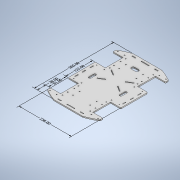
# Autodesk Inventor part: 底板2
Saved by Autodesk Inventor 2020.3 (Build 243373000, 373)
## iProperties
Created: 2020-12-02
Part Number: 底板2
Material: 常规
Document SubType Name: Sheet Metal
Designer: huang
Density: 1 g/cm^3
Sheet Metal Rule: 默认_mm
Appearance: 默认
Author: huang
Autodesk Inventor part; units mm, degrees
ref_plane "YZ Plane" through (0, 0, 0) normal (1, 0, 0) x (0, 1, 0)
ref_plane "XZ Plane" through (0, 0, 0) normal (0, 1, 0) x (-1, 0, 0)
ref_plane "XY Plane" through (0, 0, 0) normal (0, 0, 1) x (1, 0, 0)
sketch "草图1" plane through (0, 0, 0) normal (0, 1, 0) x (-1, 0, 0)
  line L0 (-53.8986, 0) -> (-183.8986, 0)
  line L1 (-237.8986, 27.6517) -> (-237.8986, 332.3483)
  line L2 (-183.8986, 360) -> (-53.8986, 360)
  line L3 (0.1014, 332.3483) -> (0.1014, 27.6517)
  arc A0 (-53.8986, 0) -> (-2.4158, 23.3117) centre (-151.1817, 283.3499) ccw
  arc A1 (-2.4158, 23.3117) -> (0.1014, 27.6517) centre (-4.8986, 27.6517) ccw
  arc A2 (-235.3815, 23.3117) -> (-183.8986, 0) centre (-86.6156, 283.3499) ccw
  arc A3 (-237.8986, 27.6517) -> (-235.3815, 23.3117) centre (-232.8986, 27.6517) ccw
  arc A4 (-2.4158, 336.6883) -> (-53.8986, 360) centre (-151.1817, 76.6501) ccw
  arc A5 (0.1014, 332.3483) -> (-2.4158, 336.6883) centre (-4.8986, 332.3483) ccw
  arc A6 (-183.8986, 360) -> (-235.3815, 336.6883) centre (-86.6156, 76.6501) ccw
  arc A7 (-235.3815, 336.6883) -> (-237.8986, 332.3483) centre (-232.8986, 332.3483) ccw
  line L4 (-118.8986, 10) -> (-135.3986, 10)
  line L5 (-118.8986, 10) -> (-102.3986, 10)
  line L6 (-102.3986, 13) -> (-135.3986, 13)
  arc A8 (-102.3986, 10) -> (-102.3986, 13) centre (-102.3986, 11.5) ccw
  arc A9 (-135.3986, 13) -> (-135.3986, 10) centre (-135.3986, 11.5) ccw
  arc A10 (-163.3986, 10) -> (-163.3986, 13) centre (-163.3986, 11.5) ccw
  line L7 (-163.3986, 10) -> (-176.3986, 10)
  line L8 (-176.3986, 13) -> (-163.3986, 13)
  arc A11 (-176.3986, 13) -> (-176.3986, 10) centre (-176.3986, 11.5) ccw
  line L9 (-118.8986, 50) -> (-127.3986, 50)
  line L10 (-118.8986, 50) -> (-110.3986, 50)
  line L11 (-110.3986, 65) -> (-127.3986, 65)
  arc A12 (-110.3986, 50) -> (-110.3986, 65) centre (-110.3986, 57.5) ccw
  arc A13 (-127.3986, 65) -> (-127.3986, 50) centre (-127.3986, 57.5) ccw
  circle A14 centre (-181.8986, 37) radius 2
  circle A15 centre (-197.8986, 26) radius 2
  circle A16 centre (-227.8986, 26) radius 2
  circle A17 centre (-181.8986, 109) radius 2
  circle A18 centre (-186.8986, 128) radius 2
  circle A19 centre (-222.3986, 128) radius 1.5
  arc A20 (-170.3606, 115.4419) -> (-168.7656, 112.901) centre (-169.5632, 114.1714) ccw
  arc A21 (-146.0526, 127.161) -> (-147.6449, 129.6982) centre (-146.7796, 128.473) ccw
  line L12 (-145.9139, 127.248) -> (-168.7656, 112.901)
  line L13 (-147.5067, 129.785) -> (-170.3606, 115.4419)
  arc A22 (-168.7665, 179.0438) -> (-170.3606, 176.5041) centre (-169.5635, 177.774) ccw
  arc A23 (-147.6449, 162.2478) -> (-146.0526, 164.785) centre (-146.7796, 163.473) ccw
  line L14 (-145.914, 164.698) -> (-168.7665, 179.0438)
  line L15 (-147.5067, 162.161) -> (-170.3606, 176.5041)
  arc A24 (-69.0307, 112.9022) -> (-67.4366, 115.4419) centre (-68.2337, 114.172) ccw
  arc A25 (-90.1523, 129.6982) -> (-91.7447, 127.161) centre (-91.0176, 128.473) ccw
  line L16 (-91.8832, 127.248) -> (-69.0307, 112.9022)
  line L17 (-90.2906, 129.785) -> (-67.4366, 115.4419)
  arc A26 (-91.7447, 164.785) -> (-90.1523, 162.2478) centre (-91.0176, 163.473) ccw
  line L18 (-90.2906, 162.161) -> (-67.4366, 176.5041)
  line L19 (-91.8832, 164.698) -> (-69.0307, 179.0438)
  arc A27 (-67.4366, 176.5041) -> (-69.0307, 179.0438) centre (-68.2337, 177.774) ccw
  arc A28 (-228.4486, 139.55) -> (-225.4486, 139.55) centre (-226.9486, 139.55) ccw
  line L20 (-225.4486, 139.55) -> (-225.4486, 151.55)
  line L21 (-228.4486, 151.55) -> (-228.4486, 139.55)
  arc A29 (-225.4486, 151.55) -> (-228.4486, 151.55) centre (-226.9486, 151.55) ccw
  arc A30 (-193.8986, 169.55) -> (-183.8986, 169.55) centre (-188.8986, 169.55) ccw
  arc A31 (-183.8986, 191.55) -> (-193.8986, 191.55) centre (-188.8986, 191.55) ccw
  line L22 (-183.8986, 191.55) -> (-183.8986, 169.55)
  line L23 (-193.8986, 169.55) -> (-193.8986, 191.55)
  arc A32 (-228.8986, 174.5) -> (-225.8986, 174.5) centre (-227.3986, 174.5) ccw
  arc A33 (-225.8986, 186.5) -> (-228.8986, 186.5) centre (-227.3986, 186.5) ccw
  line L24 (-225.8986, 174.5) -> (-225.8986, 186.5)
  line L25 (-228.8986, 186.5) -> (-228.8986, 174.5)
  arc A34 (-163.3986, 347) -> (-163.3986, 350) centre (-163.3986, 348.5) ccw
  line L26 (-163.3986, 350) -> (-176.3986, 350)
  line L27 (-176.3986, 347) -> (-163.3986, 347)
  arc A35 (-176.3986, 350) -> (-176.3986, 347) centre (-176.3986, 348.5) ccw
  circle A36 centre (-181.8986, 323) radius 2
  circle A37 centre (-197.8986, 334) radius 2
  circle A38 centre (-227.8986, 334) radius 2
  circle A39 centre (-181.8986, 251) radius 2
  circle A40 centre (-186.8986, 232) radius 2
  circle A41 centre (-222.3986, 232) radius 1.5
  arc A42 (-225.4486, 220.45) -> (-228.4486, 220.45) centre (-226.9486, 220.45) ccw
  line L28 (-225.4486, 220.45) -> (-225.4486, 208.45)
  line L29 (-228.4486, 208.45) -> (-228.4486, 220.45)
  arc A43 (-228.4486, 208.45) -> (-225.4486, 208.45) centre (-226.9486, 208.45) ccw
  line L30 (-118.8986, 350) -> (-135.3986, 350)
  line L31 (-118.8986, 350) -> (-102.3986, 350)
  line L32 (-102.3986, 347) -> (-135.3986, 347)
  arc A44 (-102.3986, 347) -> (-102.3986, 350) centre (-102.3986, 348.5) ccw
  arc A45 (-135.3986, 350) -> (-135.3986, 347) centre (-135.3986, 348.5) ccw
  arc A46 (-74.3986, 13) -> (-74.3986, 10) centre (-74.3986, 11.5) ccw
  line L33 (-74.3986, 10) -> (-61.3986, 10)
  line L34 (-61.3986, 13) -> (-74.3986, 13)
  arc A47 (-61.3986, 10) -> (-61.3986, 13) centre (-61.3986, 11.5) ccw
  circle A48 centre (-55.8986, 37) radius 2
  circle A49 centre (-39.8986, 26) radius 2
  circle A50 centre (-9.8986, 26) radius 2
  circle A51 centre (-55.8986, 109) radius 2
  circle A52 centre (-50.8986, 128) radius 2
  circle A53 centre (-15.3986, 128) radius 1.5
  arc A54 (-12.3486, 139.55) -> (-9.3486, 139.55) centre (-10.8486, 139.55) ccw
  line L35 (-12.3486, 139.55) -> (-12.3486, 151.55)
  line L36 (-9.3486, 151.55) -> (-9.3486, 139.55)
  arc A55 (-9.3486, 151.55) -> (-12.3486, 151.55) centre (-10.8486, 151.55) ccw
  arc A56 (-53.8986, 169.55) -> (-43.8986, 169.55) centre (-48.8986, 169.55) ccw
  arc A57 (-43.8986, 191.55) -> (-53.8986, 191.55) centre (-48.8986, 191.55) ccw
  line L37 (-53.8986, 191.55) -> (-53.8986, 169.55)
  line L38 (-43.8986, 169.55) -> (-43.8986, 191.55)
  arc A58 (-11.8986, 174.5) -> (-8.8986, 174.5) centre (-10.3986, 174.5) ccw
  arc A59 (-8.8986, 186.5) -> (-11.8986, 186.5) centre (-10.3986, 186.5) ccw
  line L39 (-11.8986, 174.5) -> (-11.8986, 186.5)
  line L40 (-8.8986, 186.5) -> (-8.8986, 174.5)
  circle A60 centre (-55.8986, 323) radius 2
  circle A61 centre (-39.8986, 334) radius 2
  arc A62 (-74.3986, 350) -> (-74.3986, 347) centre (-74.3986, 348.5) ccw
  line L41 (-74.3986, 350) -> (-61.3986, 350)
  line L42 (-61.3986, 347) -> (-74.3986, 347)
  arc A63 (-61.3986, 347) -> (-61.3986, 350) centre (-61.3986, 348.5) ccw
  circle A64 centre (-9.8986, 334) radius 2
  circle A65 centre (-55.8986, 251) radius 2
  circle A66 centre (-50.8986, 232) radius 2
  line L43 (-12.3486, 220.45) -> (-12.3486, 208.45)
  arc A67 (-9.3486, 220.45) -> (-12.3486, 220.45) centre (-10.8486, 220.45) ccw
  line L44 (-9.3486, 208.45) -> (-9.3486, 220.45)
  arc A68 (-12.3486, 208.45) -> (-9.3486, 208.45) centre (-10.8486, 208.45) ccw
  circle A69 centre (-15.3986, 232) radius 1.5
  dimension "d33" = 360
  dimension "d34" = 238
  dimension "d38" = 5
  dimension "d40" = 16.5
  dimension "d42" = 3
  dimension "d45" = 13
  dimension "d46" = 3
  dimension "d50" = 15
  constraints: 100 point on circle, 90 end point, 70 centre point, 11 tangent, 8 point on line, 6 horizontal, 4 parallel, 1 perpendicular
  measures "d33" distance between parallel lines of L2 L0
  measures "d34" distance between parallel lines of L1 L3
  measures "d38" radius of A1
  measures "d40" distance of L4.start L4.end
  measures "d42" distance of L5.end L6.start
  measures "d45" distance of L7.start L7.end
  measures "d46" distance of L7.end L8.start
  measures "d50" distance of L10.end L11.start
extrude "拉伸1" add sketch "草图1" along normal blind 5
sketch "草图2" plane through (0, 5, 0) normal (0, 1, 0) x (1, 0, 0)
  circle A0 centre (227.8986, -334) radius 2 projected
  line L0 (237.8986, -332.3483) -> (237.8986, -27.6517) projected
  line L1 (237.8986, -322) -> (191.8986, -322)
  line L2 (191.8986, -322) -> (191.8986, -241)
  line L3 (191.8986, -241) -> (237.8986, -241)
  line L4 (-15.016, -180) -> (322.8626, -180)
  line L5 (118.8986, -393.244) -> (118.8986, 135.9875)
  line L6 (237.8986, -38) -> (191.8986, -38)
  line L7 (191.8986, -38) -> (191.8986, -119)
  line L8 (191.8986, -119) -> (237.8986, -119)
  line L9 (-0.1014, -322) -> (45.8986, -322)
  line L10 (45.8986, -322) -> (45.8986, -241)
  line L11 (45.8986, -241) -> (-0.1014, -241)
  line L12 (-0.1014, -38) -> (45.8986, -38)
  line L13 (45.8986, -38) -> (45.8986, -119)
  line L14 (45.8986, -119) -> (-0.1014, -119)
  line L15 (237.8986, -322) -> (237.8986, -241)
  line L16 (237.8986, -119) -> (237.8986, -38)
  line L17 (-0.1014, -38) -> (-0.1014, -119)
  line L18 (-0.1014, -27.6517) -> (-0.1014, -332.3483) projected
  line L19 (-0.1014, -241) -> (-0.1014, -322)
  point P0 (0, 0)
  dimension "d97" = 81
  constraints: 36 end point, 12 symmetric about line, 4 collinear, 2 point on line, 2 vertical, 1 horizontal, 1 perpendicular
  measures "d97" distance of L1.end L2.end
extrude "拉伸2" cut sketch "草图2" against normal through all contours L1 L2 L3 L0 | L8 L7 L6 L0 | L18 L11 L10 L9 | L12 L13 L14 L17
fillet "圆角1" radius 3 8 edges at (237.8986, 2.5, 38) (237.8986, 2.5, 241) (237.8986, 2.5, 119) (237.8986, 2.5, 322) (-0.1014, 2.5, 322) (-0.1014, 2.5, 241) (-0.1014, 2.5, 119) (-0.1014, 2.5, 38)
sketch "草图3" plane through (0, 5, 0) normal (0, 1, 0) x (1, 0, 0)
  circle A0 centre (181.8986, -270) radius 2
  circle A1 centre (157.8986, -270) radius 2
  circle A2 centre (157.8986, -300) radius 2
  circle A3 centre (181.8986, -300) radius 2
  line L0 (118.8986, -378.6096) -> (118.8986, 67.6324)
  line L1 (-11.6879, -180) -> (265.2899, -180)
  circle A4 centre (181.8986, -90) radius 2
  circle A5 centre (157.8986, -90) radius 2
  circle A6 centre (157.8986, -60) radius 2
  circle A7 centre (181.8986, -60) radius 2
  circle A8 centre (55.8986, -270) radius 2
  circle A9 centre (79.8986, -270) radius 2
  circle A10 centre (79.8986, -300) radius 2
  circle A11 centre (55.8986, -300) radius 2
  circle A12 centre (55.8986, -90) radius 2
  circle A13 centre (79.8986, -90) radius 2
  circle A14 centre (79.8986, -60) radius 2
  circle A15 centre (55.8986, -60) radius 2
  point P0 (0, 0)
  dimension "d112" = 4
  dimension "d114" = 4
  constraints: 16 centre point, 12 symmetric about line, 4 end point, 1 horizontal, 1 vertical, 12 other
  measures "d112" diameter of A2
  measures "d114" diameter of A3
extrude "拉伸3" cut sketch "草图3" against normal through all
equation "\"折弯半径\" = 厚度"
equation "\"折弯释压宽度\" = 厚度"
equation "\"折弯释压深度\" = 0.5 * 厚度"
equation "\"拐角释压尺寸\" = 4 * 厚度"
equation "\"最小余量\" = 2 * 厚度"
equation "\"过渡半径\" = 折弯半径"
equation "\"Jacobi半径尺寸\" = 折弯半径"
equation "\"间隙大小\" = 厚度"
equation "\"厚度\" = 0.5"
